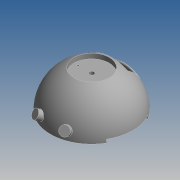
# Autodesk Inventor part: body_face
Saved by Autodesk Inventor 2017 (Build 210142000, 142)
## iProperties
Created: 2018-10-05
Part Number: body_face
Material: Générique
Document SubType Name: Modeling
Designer: Gilles Mottiez
Density: 1 g/cm^3
Appearance: Par défaut
Author: Gilles Mottiez
Autodesk Inventor part; units mm, degrees
ref_plane "YZ Plane" through (0, 0, 0) normal (1, 0, 0) x (0, 1, 0)
ref_plane "XZ Plane" through (0, 0, 0) normal (0, 1, 0) x (-1, 0, 0)
ref_plane "XY Plane" through (0, 0, 0) normal (0, 0, 1) x (1, 0, 0)
sketch "Sketch1" plane through (0, 0, 0) normal (0, 0, 1) x (1, 0, 0)
  circle A0 centre (0, 0) radius 70 construction
  line L0 (-70, 0) -> (70, 0) construction
  arc A1 (70, 0) -> (-70, 0) centre (0, 0) ccw
  line L1 (-70, 0) -> (70, 0)
  dimension "d0" = 140
  constraints: 4 end point, 4 point on circle, 2 centre point, 2 coincident, 1 collinear, 1 concentric, 1 horizontal, 1 midpoint
  measures "d0" diameter of A0
revolve "Révolution1" add sketch "Sketch1" angle 180 about axis through (-70, 0, 0) along (1, 0, 0)
sketch "Esquisse2" plane through (0, 0, 0) normal (1, 0, 0) x (0, 1, 0)
  line L0 (-70, 0) -> (70, 0) construction
  circle A0 centre (0, 0) radius 67 construction
  arc A1 (67, 0) -> (-67, 0) centre (0, 0) ccw
  line L1 (67, 0) -> (-67, 0)
  dimension "d2" = 134
  constraints: 4 point on circle, 2 centre point, 2 concentric, 2 end point, 2 point on line, 1 coincident, 1 collinear
  measures "d2" diameter of A0
revolve "Révolution2" cut sketch "Esquisse2" angle 360 about axis through (0, 67, 0) along (0, -1, 0)
sketch "Esquisse3" plane through (0, 0, 0) normal (1, 0, 0) x (0, 1, 0)
  line L0 (67, 0) -> (-67, 0) construction
  line L1 (-70, 0) -> (70, 0) construction
  arc A0 (70, 0) -> (-70, 0) centre (0, 0) ccw construction
  line L2 (35, 0) -> (-35, 0)
  line L3 (-35, 0) -> (-35, 5.5)
  line L4 (-35, 5.5) -> (35, 5.5)
  line L5 (35, 5.5) -> (35, 0)
  point P0 (0, 0)
  point P1 (0, 0)
  point P2 (0, 5.5)
  dimension "d4" = 70
  dimension "d5" = 5.5
  constraints: 8 end point, 2 midpoint, 2 parallel, 1 horizontal, 1 perpendicular, 1 point on line, 1 vertical alignment
  measures "d4" distance of L3.end L4.end
  measures "d5" distance of L4.end L2.start
extrude "Extrusion1" cut sketch "Esquisse3" along normal through all both and the other way through all
sketch "Esquisse4" plane through (0, 0, 0) normal (0, 0, -1) x (-1, 0, 0)
  line L0 (-60.6218, 35) -> (-57.1314, 35) construction
  arc A0 (57.1314, 35) -> (-57.1314, 35) centre (0, 0) ccw construction
  line L1 (57.1314, 35) -> (60.6218, 35) construction
  arc A1 (60.6218, 35) -> (-60.6218, 35) centre (0, 0) ccw construction
  arc A2 (-57.1314, -35) -> (57.1314, -35) centre (0, 0) ccw construction
  line L2 (-57.1314, -35) -> (-60.6218, -35) construction
  arc A3 (-60.6218, -35) -> (60.6218, -35) centre (0, 0) ccw construction
  line L3 (60.6218, -35) -> (57.1314, -35) construction
  arc A4 (-57.1314, -35) -> (57.1314, -35) centre (0, 0) ccw construction
  arc A5 (-56.8661, 35) -> (-56.8661, -35) centre (0, 0) ccw construction
  line L4 (-60.3718, 35) -> (-56.8661, 35) construction
  arc A6 (-60.3718, 35) -> (-60.3718, -35) centre (0, 0) ccw construction
  line L5 (-60.3718, -35) -> (-56.8661, -35) construction
  arc A7 (56.8661, -35) -> (56.8661, 35) centre (0, 0) ccw construction
  line L6 (56.8661, -35) -> (60.3718, -35) construction
  arc A8 (60.3718, -35) -> (60.3718, 35) centre (0, 0) ccw construction
  line L7 (56.8661, 35) -> (60.3718, 35) construction
  line L8 (0, 0) -> (-49.4975, 49.4975) construction
  line L9 (0, 0) -> (-69.7836, 0) construction
  circle A9 centre (0, 0) radius 63 construction
  circle A10 centre (-44.5477, 44.5477) radius 4 construction
  line L10 (-41.6309, 47.2849) -> (-44.5602, 50.0339)
  line L11 (-47.2849, 41.6309) -> (-50.2031, 44.3694)
  arc A11 (-44.5602, 50.0339) -> (-50.2031, 44.3694) centre (0, 0) ccw
  arc A12 (-47.2849, 41.6309) -> (-41.6309, 47.2849) centre (-44.5477, 44.5477) ccw
  dimension "d8" = 45
  dimension "d9" = 126
  dimension "d10" = 8
  constraints: 13 point on circle, 8 end point, 4 centre point, 2 concentric, 2 tangent, 1 coincident, 1 parallel, 1 point on line
  measures "d8" angle of L8 L9
  measures "d9" diameter of A9
  measures "d10" diameter of A10
extrude "Extrusion2" add sketch "Esquisse4" against normal up to surface
sketch "Esquisse6" plane through (0, 0, 0) normal (0, 0, -1) x (-1, 0, 0)
  line L0 (-60.6218, 35) -> (-57.1314, 35) construction
  arc A0 (-50.2031, 44.3694) -> (-57.1314, 35) centre (0, 0) ccw construction
  line L1 (-50.2031, 44.3694) -> (-47.2849, 41.6309) construction
  arc A1 (-47.2849, 41.6309) -> (-41.6309, 47.2849) centre (-44.5477, 44.5477) ccw construction
  line L2 (-41.6309, 47.2849) -> (-44.5602, 50.0339) construction
  line L3 (57.1314, 35) -> (60.6218, 35) construction
  arc A2 (60.6218, 35) -> (-60.6218, 35) centre (0, 0) ccw construction
  circle A3 centre (-44.5477, 44.5477) radius 2.5
  line L4 (-57.1314, -35) -> (-60.6218, -35) projected
  arc A4 (-60.6218, -35) -> (60.6218, -35) centre (0, 0) ccw projected
  line L5 (60.6218, -35) -> (57.1314, -35) projected
  arc A5 (-57.1314, -35) -> (57.1314, -35) centre (0, 0) ccw projected
  arc A6 (57.1314, 35) -> (-44.5602, 50.0339) centre (0, 0) ccw projected
  dimension "d19" = 5
  constraints: 1 centre point, 1 coincident
  measures "d19" diameter of A3
extrude "Extrusion4" cut sketch "Esquisse6" against normal blind 4 contours A3
sketch "Esquisse7" plane through (0, 0, 0) normal (0, 0, 1) x (1, 0, 0)
  arc A0 (-60.6218, -35) -> (60.6218, -35) centre (0, 0) ccw construction
  arc A1 (57.1314, 35) -> (50.2031, 44.3694) centre (0, 0) ccw construction
  line L0 (-57.1314, -35) -> (-56.8661, -35) construction
  arc A2 (-56.8661, 35) -> (-56.8661, -35) centre (0, 0) ccw construction
  line L1 (-56.8661, 35) -> (-57.1314, 35) construction
  line L2 (44.5602, 50.0339) -> (41.6309, 47.2849) construction
  line L3 (47.2849, 41.6309) -> (50.2031, 44.3694) construction
  line L4 (57.1314, 35) -> (56.8661, 35) construction
  arc A3 (56.8661, -35) -> (56.8661, 35) centre (0, 0) ccw construction
  line L5 (56.8661, -35) -> (57.1314, -35) construction
  line L6 (50, -70) -> (-50, -70) construction
  arc A4 (-57.1314, -35) -> (57.1314, -35) centre (0, 0) ccw projected
  arc A5 (44.5602, 50.0339) -> (-57.1314, 35) centre (0, 0) ccw projected
  point P0 (0, -70)
  point P1 (0, -70)
  dimension "d25" = 100
  constraints: 2 end point, 1 coincident, 1 horizontal, 1 midpoint, 1 point on circle, 1 vertical alignment, 1 other
  measures "d25" distance of L6.start L6.end
ref_plane "Plan de construction1" through (50, -70, 0) normal (0, -0.8660254, 0.5) x (-1, 0, 0)
ref_plane "Plan de construction2" through (50, -78.6603, 5) normal (0, -0.8660254, 0.5) x (-1, 0, 0)
sketch "Esquisse9" plane through (50, -78.6603, 5) normal (0, -0.8660254, 0.5) x (-1, 0, 0)
  line L0 (0, 0) -> (100, 0) construction
  ellipse E0 centre (50, -52.5) end of major axis (110.6218, -52.5) minor radius 52.5 (-10.6218, -52.5) -> (-10.3718, -57.2631) ccw construction
  ellipse E1 centre (50, -35) end of major axis (120, -35) minor radius 35 (-10.6218, -52.5) -> (110.6218, -52.5) ccw construction
  ellipse E2 centre (50, -52.5) end of major axis (110.6218, -52.5) minor radius 52.5 (110.3718, -57.2631) -> (110.6218, -52.5) ccw construction
  ellipse E3 centre (50, -39.7631) end of major axis (119.7836, -39.7631) minor radius 34.8918 (110.3718, -57.2631) -> (110.3718, -22.2631) ccw construction
  ellipse E4 centre (50, -17.5) end of major axis (110.6218, -17.5) minor radius 52.5 (110.3718, -22.2631) -> (110.6218, -17.5) ccw construction
  ellipse E5 centre (50, -35) end of major axis (120, -35) minor radius 35 (110.6218, -17.5) -> (-10.6218, -17.5) ccw construction
  ellipse E6 centre (50, -17.5) end of major axis (110.6218, -17.5) minor radius 52.5 (-10.6218, -17.5) -> (-10.3718, -22.2631) ccw construction
  ellipse E7 centre (50, -39.7631) end of major axis (119.7836, -39.7631) minor radius 34.8918 (-10.3718, -22.2631) -> (-10.3718, -57.2631) ccw construction
  line L1 (75, 0) -> (75, -50) construction
  line L2 (25, 0) -> (25, -50) construction
  point P0 (50, -35)
  point P1 (50, 0)
  dimension "d32" = 50
  dimension "d34" = 25
  dimension "d40" = 50
  dimension "d41" = 25
  constraints: 4 end point, 2 point on line, 2 vertical, 8 other
  measures "d32" distance of L1.start L1.end
  measures "d34" distance from line of point (50, 0) L1
  measures "d40" distance of L2.start L2.end
  measures "d41" distance from line of L2 point (50, -17.5)
ref_plane "Plan de construction3" through (-25, -78.6603, 5) normal (-0.3420201, -0.8137977, 0.4698463) x (0, 0.5, 0.8660254)
sketch "Esquisse10" plane through (-25, -78.6603, 5) normal (-0.3420201, -0.8137977, 0.4698463) x (0, 0.5, 0.8660254)
  ellipse E0 centre (52.5, 11.0287) end of major axis (21.6025, 63.1856) minor radius 49.3339 (52.5, -45.9371) -> (57.2631, -46.6428) ccw construction
  ellipse E1 centre (35, 0.6618) end of major axis (48.5607, 69.3357) minor radius 32.8892 (52.5, -45.9371) -> (52.5, 67.9945) ccw construction
  ellipse E2 centre (52.5, 11.0287) end of major axis (21.6025, 63.1856) minor radius 49.3339 (57.2631, 66.819) -> (52.5, 67.9945) ccw construction
  ellipse E3 centre (39.7631, -0.2788) end of major axis (53.2819, 68.1828) minor radius 32.7876 (57.2631, 66.819) -> (22.2631, 46.0852) ccw construction
  ellipse E4 centre (17.5, -9.7052) end of major axis (-13.3975, 42.4517) minor radius 49.3339 (22.2631, 46.0852) -> (17.5, 47.2607) ccw construction
  ellipse E5 centre (35, 0.6618) end of major axis (48.5607, 69.3357) minor radius 32.8892 (17.5, 47.2607) -> (17.5, -66.671) ccw construction
  ellipse E6 centre (17.5, -9.7052) end of major axis (-13.3975, 42.4517) minor radius 49.3339 (17.5, -66.671) -> (22.2631, -67.3766) ccw construction
  ellipse E7 centre (39.7631, -0.2788) end of major axis (53.2819, 68.1828) minor radius 32.7876 (22.2631, -67.3766) -> (57.2631, -46.6428) ccw construction
  line L0 (0, 0) -> (50, 0) construction
  line L1 (0, -70.4769) -> (0, 23.4923) construction
  circle A0 centre (15, 0) radius 7.5
  point P0 (35, 0.6618)
  dimension "d36" = 15
  dimension "d37" = 15
  constraints: 1 centre point, 1 point on line, 8 other
  measures "d36" diameter of A0
  measures "d37" distance from line of L1 A0.centre
extrude "Extrusion5" add sketch "Esquisse10" against normal up to surface
ref_plane "Plan de construction4" through (25, -78.6603, 5) normal (0.3420201, -0.8137977, 0.4698463) x (0, 0.5, 0.8660254)
sketch "Esquisse11" plane through (25, -78.6603, 5) normal (0.3420201, -0.8137977, 0.4698463) x (0, 0.5, 0.8660254)
  line L0 (0, 0) -> (50, 0) construction
  line L1 (0, -23.4923) -> (0, 70.4769) construction
  circle A0 centre (15, 0) radius 7.5
  point P0 (35, -0.6618)
  dimension "d43" = 15
  dimension "d44" = 15
  constraints: 1 centre point, 1 point on line
  measures "d43" diameter of A0
  measures "d44" distance from line of L1 A0.centre
extrude "Extrusion6" add sketch "Esquisse11" against normal up to surface
sketch "Esquisse12" plane through (0, 0, 0) normal (1, 0, 0) x (0, 1, 0)
  arc A0 (67, 0) -> (-67, 0) centre (0, 0) ccw construction
  arc A1 (70, 0) -> (-70, 0) centre (0, 0) ccw construction
  line L0 (0, -14.3596) -> (0, 86.1577) construction
  line L1 (35, 0) -> (44.3694, 0) construction
  line L2 (-35, 0) -> (-35, 5.5) construction
  line L3 (-35, 5.5) -> (35, 5.5) construction
  line L4 (35, 5.5) -> (35, 0) construction
  ellipse E0 centre (4.3693, 0) end of major axis (4.3693, -66.7315) minor radius 45.6646 (50.0339, 0) -> (47.2849, 22.8035) ccw construction
  ellipse E1 centre (-1.4584, 0) end of major axis (-1.4584, 66.9701) minor radius 45.8278 (44.3694, 0) -> (41.6309, 22.8035) ccw construction
  line L5 (35, 0) -> (35, 5.5) construction
  line L6 (35, 5.5) -> (-35, 5.5) construction
  line L7 (-35, 5.5) -> (-35, 0) construction
  line L8 (0, 47) -> (47.7493, 47)
  arc A2 (47.7493, 47) -> (0, 67) centre (0, 0) ccw
  line L9 (0, 67) -> (0, 47)
  line L10 (-35, 0) -> (-35, 0) projected
  line L11 (50.0339, 0) -> (35, 0) projected
  point P0 (0, 0)
  point P1 (4, 66.8805)
  point P2 (-4, 66.8805)
  dimension "d48" = 20
  constraints: 4 end point, 4 point on circle, 2 point on line, 1 centre point, 1 collinear, 1 concentric, 1 horizontal, 1 horizontal alignment, 2 other
  measures "d48" distance from line of L9.start L8
revolve "Révolution3" add sketch "Esquisse12" angle 360 about axis through (0, 0, 67) along (0, 0, -1)
sketch "Esquisse13" plane through (0, 0, 0) normal (1, 0, 0) x (0, 1, 0)
  line L0 (35, 5.5) -> (35, 0) construction
  line L1 (35, 0) -> (35, 0) construction
  line L2 (35, 0) -> (35, 5.5) construction
  line L3 (35, 5.5) -> (-35, 5.5) construction
  line L4 (-35, 5.5) -> (-35, 0) construction
  line L5 (-35, 0) -> (-35, 0) construction
  line L6 (-35, 0) -> (-35, 5.5) construction
  line L7 (-35, 5.5) -> (35, 5.5) construction
  line L8 (47.7493, 47) -> (-47.7493, 47) construction
  line L9 (0, -15) -> (0, 90) construction
  arc A0 (70, 0) -> (-70, 0) centre (0, 0) ccw construction
  line L10 (0, 55) -> (30, 55) construction
  line L11 (30, 55) -> (30, 75) construction
  line L12 (30, 75) -> (0, 75) construction
  line L13 (0, 75) -> (0, 55) construction
  line L14 (0, 55) -> (30, 55)
  line L15 (30, 55) -> (30, 63.2456)
  arc A1 (30, 63.2456) -> (0, 70) centre (0, 0) ccw
  line L16 (0, 55) -> (0, 70)
  point P0 (0, 0)
  dimension "d50" = 8
  dimension "d51" = 30
  dimension "d52" = 20
  constraints: 14 end point, 4 point on circle, 3 point on line, 2 collinear, 2 parallel, 1 centre point, 1 concentric, 1 horizontal, 1 perpendicular, 2 other
  measures "d50" distance between parallel lines of L10 L8
  measures "d51" distance between parallel lines of L13 L11
  measures "d52" distance of L10.end L11.end
revolve "Révolution4" cut sketch "Esquisse13" angle 360 about axis through (0, 0, 55) along (0, 0, 1)
sketch "Esquisse15" plane through (0, 0, 55) normal (0, 0, 1) x (1, 0, 0)
  point P0 (0, 0)
  point P1 (-23, 0)
  dimension "d57" = 23
  constraints: 1 horizontal alignment
  measures "d57" distance of point (-23, 0) point (0, 0)
hole "Perçage1" at (-23, 0, 55) direction (0, 0, -1) diameter 3 depth 8 tip angle 118
sketch "Esquisse16" plane through (0, 0, 0) normal (1, 0, 0) x (0, 1, 0)
  line L0 (-30, 63.2456) -> (30, 63.2456) construction
  line L1 (35, 5.5) -> (35, 0) construction
  line L2 (35, 0) -> (35, 0) construction
  line L3 (35, 0) -> (35, 5.5) construction
  line L4 (35, 5.5) -> (-35, 5.5) construction
  line L5 (-35, 5.5) -> (-35, 0) construction
  line L6 (-35, 0) -> (-35, 0) construction
  line L7 (-35, 0) -> (-35, 5.5) construction
  line L8 (-35, 5.5) -> (35, 5.5) construction
  line L9 (47.7493, 47) -> (-47.7493, 47) construction
  line L10 (4, 47) -> (-4, 47) construction
  line L11 (-4, 55) -> (4, 55) construction
  line L12 (0, -13.1244) -> (0, 78.7461) construction
  line L13 (0, 41) -> (6, 41) construction
  line L14 (6, 41) -> (6, 47) construction
  line L15 (6, 47) -> (0, 47) construction
  line L16 (0, 47) -> (0, 41) construction
  arc A0 (11, 47) -> (6, 42) centre (11, 42) ccw construction
  line L17 (0, 47) -> (11, 47)
  line L18 (6, 41) -> (0, 41)
  line L19 (6, 41) -> (6, 42)
  arc A1 (11, 47) -> (6, 42) centre (11, 42) ccw
  line L20 (0, 41) -> (0, 47)
  point P0 (0, 0)
  dimension "d65" = 12
  dimension "d67" = 5
  dimension "d68" = 6
  constraints: 16 end point, 4 collinear, 4 point on circle, 4 point on line, 3 tangent, 2 centre point, 2 parallel, 1 concentric, 1 horizontal, 1 perpendicular, 2 other
  measures "d65" diameter of L14 L20
  measures "d67" radius of A0
  measures "d68" distance between parallel lines of L17 L13
revolve "Révolution5" add sketch "Esquisse16" angle 360 about axis through (0, 0, 41) along (0, 0, 1)
sketch "Esquisse17" plane through (0, 0, 41) normal (0, 0, -1) x (-1, 0, 0)
  circle A0 centre (0, 0) radius 4
  point P0 (0, 0)
  dimension "d70" = 8
  constraints: 1 centre point, 1 coincident
  measures "d70" diameter of A0
extrude "Extrusion8" cut sketch "Esquisse17" against normal through all
ref_plane "Plan de construction5" through (0, 0, 65) normal (0, 0, 1) x (1, 0, 0)
sketch "Esquisse24" plane through (0, 0, 65) normal (0, 0, 1) x (1, 0, 0)
  circle A0 centre (0, 0) radius 47.7493 construction
  circle A1 centre (0, 0) radius 30 construction
  line L0 (60.3718, 35) -> (60.6218, 35) construction
  arc A2 (60.6218, 35) -> (-60.6218, 35) centre (0, 0) ccw construction
  line L1 (-60.6218, 35) -> (-60.3718, 35) construction
  arc A3 (-60.3718, 35) -> (-60.3718, -35) centre (0, 0) ccw construction
  line L2 (-60.3718, -35) -> (-60.6218, -35) construction
  arc A4 (-60.6218, -35) -> (60.6218, -35) centre (0, 0) ccw construction
  line L3 (60.6218, -35) -> (60.3718, -35) construction
  arc A5 (60.3718, -35) -> (60.3718, 35) centre (0, 0) ccw construction
  line L4 (0, 0) -> (0, 70) construction
  line L5 (-25.5, 54) -> (25.5, 54)
  line L6 (25.5, 54) -> (25.5, 35)
  line L7 (25.5, 35) -> (-25.5, 35)
  line L8 (-25.5, 35) -> (-25.5, 54)
  point P0 (0, 0)
  dimension "d96" = 51
  dimension "d97" = 19
  dimension "d98" = 35
  constraints: 10 end point, 2 parallel, 1 horizontal, 1 perpendicular, 1 point on circle, 3 other
  measures "d96" distance of L6.end L7.end
  measures "d97" distance of L5.end L6.end
  measures "d98" distance from line of point (0, 0) L7
extrude "Extrusion12" cut sketch "Esquisse24" against normal through all
ref_plane "Plan de construction6" through (0, 0, 23) normal (0, 0, -1) x (-1, 0, 0)
sketch "Esquisse26" plane through (0, 0, 23) normal (0, 0, -1) x (-1, 0, 0)
  arc A0 (-50.2031, 44.3694) -> (-57.1314, 35) centre (0, 0) ccw construction
  line L0 (57.1314, -35) -> (56.8661, -35) construction
  arc A1 (56.8661, -35) -> (56.8661, 35) centre (0, 0) ccw construction
  line L1 (56.8661, 35) -> (57.1314, 35) construction
  line L2 (-44.5602, 50.0339) -> (-41.6309, 47.2849) construction
  line L3 (-47.2849, 41.6309) -> (-50.2031, 44.3694) construction
  line L4 (-57.1314, 35) -> (-56.8661, 35) construction
  arc A2 (-56.8661, 35) -> (-56.8661, -35) centre (0, 0) ccw construction
  line L5 (-56.8661, -35) -> (-57.1314, -35) construction
  line L6 (-25.5, 40.3702) -> (-25.5, 54) construction
  line L7 (-25.5, 54) -> (25.5, 54) construction
  line L8 (25.5, 54) -> (25.5, 40.3702) construction
  arc A3 (-25.5, 40.3702) -> (25.5, 40.3702) centre (0, 0) ccw construction
  line L9 (-25.5, 35) -> (-25.5, 40.3702) construction
  arc A4 (-25.5, 40.3702) -> (25.5, 40.3702) centre (0, 0) ccw construction
  line L10 (25.5, 40.3702) -> (25.5, 35) construction
  line L11 (25.5, 35) -> (-25.5, 35) construction
  circle A5 centre (23, 0) radius 1.5 construction
  circle A6 centre (0, 0) radius 11 construction
  line L12 (-25.5, 54) -> (25.5, 54) construction
  line L13 (25.5, 54) -> (25.5, 35) construction
  line L14 (25.5, 35) -> (-25.5, 35) construction
  line L15 (-25.5, 35) -> (-25.5, 54) construction
  line L16 (-25.5, 58) -> (25.5, 58) construction
  line L17 (25.5, 58) -> (25.5, 31) construction
  line L18 (25.5, 31) -> (-25.5, 31) construction
  line L19 (-25.5, 31) -> (-25.5, 58) construction
  line L20 (-25.5, 58) -> (-27.5, 58) construction
  line L21 (-27.5, 58) -> (-27.5, 31) construction
  line L22 (-27.5, 31) -> (-25.5, 31) construction
  line L23 (-25.5, 31) -> (-25.5, 58) construction
  line L24 (25.5, 58) -> (27.5, 58) construction
  line L25 (27.5, 58) -> (27.5, 31) construction
  line L26 (27.5, 31) -> (25.5, 31) construction
  line L27 (25.5, 31) -> (25.5, 58) construction
  line L28 (-27.5, 58) -> (27.5, 58)
  line L29 (27.5, 58) -> (27.5, 31)
  line L30 (27.5, 31) -> (-27.5, 31)
  line L31 (-27.5, 31) -> (-27.5, 58)
  line L32 (-25.5, 54) -> (25.5, 54)
  line L33 (25.5, 54) -> (25.5, 35)
  line L34 (25.5, 35) -> (-25.5, 35)
  line L35 (-25.5, 35) -> (-25.5, 54)
  arc A7 (-57.1314, -35) -> (57.1314, -35) centre (0, 0) ccw projected
  arc A8 (57.1314, 35) -> (-44.5602, 50.0339) centre (0, 0) ccw projected
  dimension "d102" = 27
  dimension "d103" = 51
  dimension "d104" = 4
  dimension "d105" = 2
  dimension "d106" = 2
  constraints: 48 end point, 12 parallel, 6 horizontal, 6 perpendicular, 1 coincident, 1 point on line, 1 vertical alignment, 1 other
  measures "d102" distance between parallel lines of L18 L16
  measures "d103" distance between parallel lines of L17 L19
  measures "d104" distance between parallel lines of L18 L11
  measures "d105" distance of L22.end L21.end
  measures "d106" distance of L25.end L26.end
extrude "Extrusion13" add sketch "Esquisse26" against normal up to next
sketch "Esquisse27" plane through (0, 0, 23) normal (0, 0, -1) x (-1, 0, 0)
  line L0 (-25.5, 35) -> (-25.5, 54) construction
  line L1 (-25.5, 54) -> (25.5, 54) construction
  line L2 (25.5, 54) -> (25.5, 35) construction
  line L3 (25.5, 35) -> (-25.5, 35) construction
  arc A0 (27.5, 56.6017) -> (24.4131, 58) centre (0, 0) ccw construction
  line L4 (-24.4131, 58) -> (24.4131, 58) construction
  arc A1 (-24.4131, 58) -> (-27.5, 56.6017) centre (0, 0) ccw construction
  line L5 (-27.5, 31) -> (-27.5, 56.6017) construction
  line L6 (27.5, 31) -> (-27.5, 31) construction
  line L7 (27.5, 56.6017) -> (27.5, 31) construction
  line L8 (-21.9, 56) -> (21.9, 56) construction
  line L9 (21.9, 56) -> (21.9, 33) construction
  line L10 (21.9, 33) -> (-21.9, 33) construction
  line L11 (-21.9, 33) -> (-21.9, 56) construction
  line L12 (-25.5, 44.5) -> (25.5, 44.5) construction
  line L13 (0, 0) -> (0, 54) construction
  point P0 (0, 0)
  dimension "d109" = 23
  dimension "d110" = 43.8
  constraints: 12 end point, 4 coincident, 3 midpoint, 2 parallel, 1 horizontal, 1 perpendicular, 2 other
  measures "d109" distance between parallel lines of L10 L8
  measures "d110" distance of L9.end L10.end
hole "Perçage2" at (21.9, 56, 23) at (-21.9, 56, 23) at (-21.9, 33, 23) at (21.9, 33, 23) direction (0, 0, 1) diameter 2 depth 5 tip angle 118
fillet "Congé2" radius 1 4 edges at (0, 54, 44.5421) (-25.5, 45.4489, 46.7349) (0, 35, 60.6218) (25.5, 45.4489, 46.7349)
mirror "Symétrie1" about plane through (0, 0, 0) normal (1, 0, 0) of "Extrusion2", "Extrusion4"
sketch "Esquisse28" plane through (0, 0, 0) normal (0, 0, -1) x (-1, 0, 0)
  line L0 (-57.1314, -35) -> (-60.6218, -35) construction
  arc A0 (-60.6218, -35) -> (60.6218, -35) centre (0, 0) ccw construction
  line L1 (60.6218, -35) -> (57.1314, -35) construction
  arc A1 (-57.1314, -35) -> (57.1314, -35) centre (0, 0) ccw construction
  line L2 (41.6309, 47.2849) -> (44.5602, 50.0339) construction
  arc A2 (44.5602, 50.0339) -> (-44.5602, 50.0339) centre (0, 0) ccw construction
  line L3 (-44.5602, 50.0339) -> (-41.6309, 47.2849) construction
  line L4 (-47.2849, 41.6309) -> (-50.2031, 44.3694) construction
  arc A3 (-50.2031, 44.3694) -> (-57.1314, 35) centre (0, 0) ccw construction
  line L5 (-57.1314, 35) -> (-56.8661, 35) construction
  arc A4 (-56.8661, 35) -> (-56.8661, -35) centre (0, 0) ccw construction
  line L6 (-56.8661, -35) -> (-57.1314, -35) construction
  arc A5 (-57.1314, -35) -> (57.1314, -35) centre (0, 0) ccw construction
  line L7 (57.1314, -35) -> (56.8661, -35) construction
  arc A6 (56.8661, -35) -> (56.8661, 35) centre (0, 0) ccw construction
  line L8 (56.8661, 35) -> (57.1314, 35) construction
  arc A7 (57.1314, 35) -> (50.2031, 44.3694) centre (0, 0) ccw construction
  line L9 (50.2031, 44.3694) -> (47.2849, 41.6309) construction
  line L10 (27.5, 56.6017) -> (27.5, 39.0352) construction
  arc A8 (-27.5, 39.0352) -> (27.5, 39.0352) centre (0, 0) ccw construction
  line L11 (-27.5, 39.0352) -> (-27.5, 56.6017) construction
  arc A9 (-24.4131, 58) -> (-27.5, 56.6017) centre (0, 0) ccw construction
  line L12 (-24.4131, 58) -> (24.4131, 58) construction
  arc A10 (27.5, 56.6017) -> (24.4131, 58) centre (0, 0) ccw construction
  line L13 (0, 0) -> (-35, -60.6218) construction
  line L14 (0, 0) -> (-66.7739, 0) construction
  circle A11 centre (0, 0) radius 63 construction
  circle A12 centre (-31.5, -54.5596) radius 4 construction
  line L15 (-34.8989, -52.4506) -> (-37.0088, -55.8511) construction
  line L16 (-27.9742, -56.4486) -> (-29.8641, -59.9761) construction
  line L17 (-37.0088, -55.8511) -> (-34.8989, -52.4506)
  line L18 (-27.9742, -56.4486) -> (-29.8641, -59.9761)
  arc A13 (-27.9742, -56.4486) -> (-34.8989, -52.4506) centre (-31.5, -54.5596) ccw
  arc A14 (-37.0088, -55.8511) -> (-29.8641, -59.9761) centre (0, 0) ccw
  arc A15 (-57.1314, -35) -> (57.1314, -35) centre (0, 0) ccw projected
  dimension "d119" = 60
  dimension "d120" = 126
  dimension "d121" = 8
  constraints: 15 point on circle, 12 end point, 4 centre point, 4 tangent, 2 collinear, 2 concentric, 1 coincident, 1 point on line, 2 other
  measures "d119" angle of L13 L14
  measures "d120" diameter of A11
  measures "d121" diameter of A12
extrude "Extrusion14" add sketch "Esquisse28" against normal up to surface
sketch "Esquisse29" plane through (0, 0, 0) normal (0, 0, -1) x (-1, 0, 0)
  line L0 (-57.1314, -35) -> (-60.6218, -35) construction
  arc A0 (-60.6218, -35) -> (60.6218, -35) centre (0, 0) ccw construction
  line L1 (60.6218, -35) -> (57.1314, -35) construction
  arc A1 (-29.8641, -59.9761) -> (57.1314, -35) centre (0, 0) ccw construction
  line L2 (-29.8641, -59.9761) -> (-27.9742, -56.4486) construction
  arc A2 (-27.9742, -56.4486) -> (-34.8989, -52.4506) centre (-31.5, -54.5596) ccw construction
  line L3 (-34.8989, -52.4506) -> (-37.0088, -55.8511) construction
  arc A3 (-57.1314, -35) -> (-37.0088, -55.8511) centre (0, 0) ccw construction
  circle A4 centre (-31.5, -54.5596) radius 2.5
  dimension "d124" = 5
  constraints: 1 centre point, 1 coincident
  measures "d124" diameter of A4
extrude "Extrusion15" cut sketch "Esquisse29" against normal blind 4
mirror "Symétrie2" about plane through (0, 0, 0) normal (1, 0, 0) of "Extrusion14", "Extrusion15"
